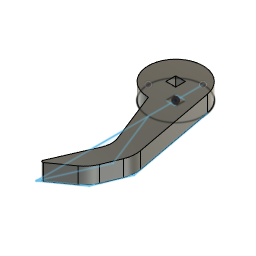
PWP Thumb (Autodesk Fusion 360 design; units mm, degrees)
Autodesk Fusion 360 part; units mm, degrees
sketch "Sketch1" plane through (0, 0, 0) normal (0, 0, 1) x (1, 0, 0)
  circle A0 centre (0, 0) radius 10
  line L0 (-1.778, 1.778) -> (1.778, 1.778)
  line L1 (1.778, 1.778) -> (1.778, -1.778)
  line L2 (1.778, -1.778) -> (-1.778, -1.778)
  line L3 (-1.778, -1.778) -> (-1.778, 1.778)
  line L4 (-1.778, 1.778) -> (1.778, -1.778) construction
  line L5 (1.778, 1.778) -> (-1.778, -1.778) construction
  line L6 (0, 10) -> (0, -50.96)
  line L7 (0, -50.96) -> (11.2783, -42.9344)
  line L8 (0, -50.96) -> (8.4708, -31.4235)
  line L9 (9.8281, 1.8461) -> (16.0511, -31.2832)
  line L10 (11.2783, -42.9344) -> (16.0511, -31.2832)
  line L11 (8.4708, -31.4235) -> (0, -10)
  point P0 (-10, 0)
  point P1 (0, 10)
  dimension "d1" = 20
  dimension "d5" = 3.556
  dimension "d14" = 60.96
  constraint coincident A0.centre origin
  constraint coincident A0 P0
  constraint horizontal L0
  constraint perpendicular L0 L1
  constraint parallel L0 L2
  constraint parallel L1 L3
  constraint coincident L4 A0.centre
  constraint coincident L5 A0.centre
  constraint coincident A0 P1
  constraint coincident P1 L6.start
  constraint perpendicular L2 L6
  constraint coincident A0 L9.start
  constraint tangent A0 L9
  constraint coincident A0 L11.end
  constraint coincident L6 L11.end
  measures "d1" diameter of A0
  measures "d5" distance of L0.start L0.end
  measures "d14" distance of P1 L6.end
extrude "Extrude1" add sketch "Sketch1" along normal blind 6 contours A0 L0 L1 L2 L6 | A0 L7 L8 L9 L10 L11 | A0 L0 L2 L3 L6
fillet "Fillet4" radius 7.5 1 edges at (8.4708, -31.4235, 3)
fillet "Fillet5" radius 10 2 edges at (16.0511, -31.2832, 3) (11.2783, -42.9344, 3)
fillet "Fillet6" radius 0.5 1 edges at (0, -50.96, 3)
